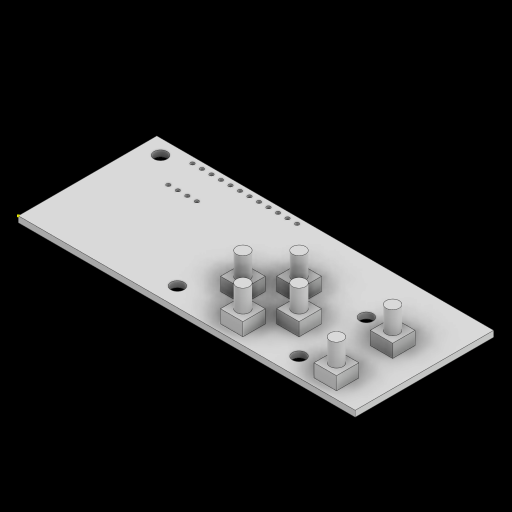
# Autodesk Inventor part: 110_PICO_Daughterboard
Saved by Autodesk Inventor 2024 (Build 280153000, 153)
## iProperties
Created: 2023-07-20
Part Number: 110_PICO_Daughterboard
Material: Generisch
Document SubType Name: Modeling
Designer: Philipp
Density: 1 g/cm^3
Appearance: Vorgabe
Author: Philipp
Autodesk Inventor part; units mm, degrees
ref_plane "YZ Plane" through (0, 0, 0) normal (1, 0, 0) x (0, 1, 0)
ref_plane "XZ Plane" through (0, 0, 0) normal (0, 1, 0) x (-1, 0, 0)
ref_plane "XY Plane" through (0, 0, 0) normal (0, 0, 1) x (1, 0, 0)
sketch "Skizze1" plane through (0, 0, 0) normal (0, 0, 1) x (1, 0, 0)
  line L0 (0, 0) -> (90, 0)
  line L1 (90, 0) -> (90, 37)
  line L2 (90, 37) -> (0, 37)
  line L3 (0, 37) -> (0, 0)
  dimension "d0" = 90
  dimension "d1" = 37
  constraints: 8 end point, 2 parallel, 1 horizontal, 1 perpendicular
  measures "d0" distance of L2.end L1.end
  measures "d1" distance of L1.end L0.end
extrude "Extrusion1" add sketch "Skizze1" against normal blind 1.6
sketch "Skizze2" plane through (0, 0, 0) normal (0, 0, 1) x (1, 0, 0)
  circle A0 centre (5, 33) radius 1.75
  circle A1 centre (37.5, 5) radius 1.75
  circle A2 centre (70, 5) radius 1.75
  circle A3 centre (70, 23) radius 1.75
  line L0 (0, 0) -> (90, 0) projected
  line L1 (0, 37) -> (0, 0) projected
  line L2 (90, 0) -> (90, 37) projected
  dimension "d4" = 3.5
  dimension "d5" = 3.5
  dimension "d6" = 3.5
  dimension "d7" = 3.5
  dimension "d8" = 33
  dimension "d9" = 5
  dimension "d10" = 37.5
  dimension "d11" = 5
  dimension "d12" = 5
  dimension "d14" = 70
  dimension "d15" = 70
  dimension "d16" = 23
  constraints: 4 centre point
  measures "d4" diameter of A0
  measures "d5" diameter of A1
  measures "d6" diameter of A2
  measures "d7" diameter of A3
  measures "d8" distance from line of L0 A0.centre
  measures "d9" distance from line of L1 A0.centre
  measures "d10" distance from line of L1 A1.centre
  measures "d11" distance from line of L0 A1.centre
  measures "d12" distance from line of L0 A2.centre
  measures "d14" distance from line of L1 A2.centre
  measures "d15" distance from line of L1 A3.centre
  measures "d16" distance from line of L0 A3.centre
extrude "Extrusion2" cut sketch "Skizze2" against normal blind 1.6
sketch "Skizze3" plane through (0, 0, 0) normal (0, 0, 1) x (1, 0, 0)
  circle A0 centre (11.152, 35.373) radius 0.5
  line L0 (0, 0) -> (90, 0) projected
  line L1 (0, 37) -> (0, 0) projected
  circle A1 centre (12.889, 27.192) radius 0.5
  dimension "d19" = 1
  dimension "d20" = 35.373
  dimension "d21" = 11.152
  dimension "d22" = 1
  dimension "d23" = 27.192
  dimension "d24" = 12.889
  constraints: 2 centre point
  measures "d19" diameter of A0
  measures "d20" distance from line of L0 A0.centre
  measures "d21" distance from line of L1 A0.centre
  measures "d22" diameter of A1
  measures "d23" distance from line of L0 A1.centre
  measures "d24" distance from line of L1 A1.centre
extrude "Extrusion3" cut sketch "Skizze3" against normal blind 1.6
pattern_linear "Rechteckige Anordnung1" count 12 spacing 2.54 along (1, 0, 0) of "Extrusion3"
sketch "Skizze4" plane through (0, 0, 0) normal (0, 0, 1) x (1, 0, 0)
  line L0 (21.549, 28.192) -> (42.329, 28.192)
  line L1 (42.329, 28.192) -> (42.329, 26.192)
  line L2 (42.329, 26.192) -> (21.549, 26.192)
  line L3 (21.549, 26.192) -> (21.549, 28.192)
  circle A0 centre (23.049, 27.192) radius 0.5 projected
  circle A1 centre (40.829, 27.192) radius 0.5 projected
  point P0 (0, 0)
  dimension "d30" = 1
  dimension "d31" = 1
  dimension "d32" = 1
  dimension "d33" = 1
  constraints: 8 end point, 2 parallel, 1 horizontal, 1 perpendicular
  measures "d30" distance edge to line of A0 L3
  measures "d31" distance edge to line of A1 L1
  measures "d32" distance from line of A0.centre L2
  measures "d33" distance from line of L0 A0.centre
extrude "Extrusion4" add sketch "Skizze4" against normal blind 1.6 contours L0 L1 L2 L3 | A0 | A1
sketch "Skizze5" plane through (0, 0, 0) normal (0, 0, 1) x (1, 0, 0)
  line L0 (0, 37) -> (0, 0) projected
  line L1 (44.5, 15.5) -> (50.5, 15.5)
  line L2 (50.5, 15.5) -> (50.5, 9.5)
  line L3 (50.5, 9.5) -> (44.5, 9.5)
  line L4 (44.5, 9.5) -> (44.5, 15.5)
  line L5 (0, 0) -> (90, 0) projected
  line L6 (52, 23) -> (58, 23)
  line L7 (58, 23) -> (58, 17)
  line L8 (58, 17) -> (52, 17)
  line L9 (52, 17) -> (52, 23)
  line L10 (52, 8) -> (58, 8)
  line L11 (58, 8) -> (58, 2)
  line L12 (58, 2) -> (52, 2)
  line L13 (52, 2) -> (52, 8)
  line L14 (59.5, 15.5) -> (65.5, 15.5)
  line L15 (65.5, 15.5) -> (65.5, 9.5)
  line L16 (65.5, 9.5) -> (59.5, 9.5)
  line L17 (59.5, 9.5) -> (59.5, 15.5)
  line L18 (77, 23) -> (83, 23)
  line L19 (83, 23) -> (83, 17)
  line L20 (83, 17) -> (77, 17)
  line L21 (77, 17) -> (77, 23)
  line L22 (77, 8) -> (83, 8)
  line L23 (83, 8) -> (83, 2)
  line L24 (83, 2) -> (77, 2)
  line L25 (77, 2) -> (77, 8)
  point P0 (44.5, 12.5)
  point P1 (47.5, 9.5)
  point P2 (55, 17)
  point P3 (52, 20)
  point P4 (52, 5)
  point P5 (55, 2)
  point P6 (62.5, 9.5)
  point P7 (59.5, 12.5)
  point P8 (83, 20)
  point P9 (80, 17)
  point P10 (83, 5)
  point P11 (80, 2)
  dimension "d34" = 1.6
  dimension "d53" = 6
  dimension "d54" = 6
  dimension "d55" = 12.5
  dimension "d56" = 47.5
  dimension "d57" = 6
  dimension "d58" = 6
  dimension "d59" = 55
  dimension "d60" = 20
  dimension "d61" = 6
  dimension "d62" = 6
  dimension "d63" = 5
  dimension "d64" = 55
  dimension "d65" = 6
  dimension "d66" = 6
  dimension "d67" = 62.5
  dimension "d68" = 12.5
  dimension "d69" = 6
  dimension "d70" = 6
  dimension "d71" = 20
  dimension "d72" = 80
  dimension "d73" = 6
  dimension "d74" = 6
  dimension "d75" = 5
  dimension "d76" = 80
  constraints: 48 end point, 12 midpoint, 12 parallel, 6 horizontal, 6 perpendicular
  measures "d53" distance of L2.end L3.end
  measures "d54" distance of L1.end L2.end
  measures "d55" distance from line of L5 point (44.5, 12.5)
  measures "d56" distance from line of point (47.5, 9.5) L0
  measures "d57" distance of L7.end L8.end
  measures "d58" distance of L6.end L7.end
  measures "d59" distance from line of L0 point (55, 17)
  measures "d60" distance from line of L5 point (52, 20)
  measures "d61" distance of L11.end L12.end
  measures "d62" distance of L10.end L11.end
  measures "d63" distance from line of L5 point (52, 5)
  measures "d64" distance from line of L0 point (55, 2)
  measures "d65" distance of L15.end L16.end
  measures "d66" distance of L14.end L15.end
  measures "d67" distance from line of L0 point (62.5, 9.5)
  measures "d68" distance from line of L5 point (59.5, 12.5)
  measures "d69" distance of L19.end L20.end
  measures "d70" distance of L18.end L19.end
  measures "d71" distance from line of L5 point (83, 20)
  measures "d72" distance from line of L0 point (80, 17)
  measures "d73" distance of L23.end L24.end
  measures "d74" distance of L22.end L23.end
  measures "d75" distance from line of L5 point (83, 5)
  measures "d76" distance from line of L0 point (80, 2)
extrude "Extrusion5" add sketch "Skizze5" along normal blind 3.5
sketch "Skizze6" plane through (0, 0, 3.5) normal (0, 0, 1) x (1, 0, 0)
  line L0 (52, 17) -> (58, 17) projected
  line L1 (58, 17) -> (58, 23) projected
  line L2 (58, 23) -> (52, 23) projected
  line L3 (52, 23) -> (52, 17) projected
  line L4 (44.5, 9.5) -> (50.5, 9.5) projected
  line L5 (50.5, 9.5) -> (50.5, 15.5) projected
  line L6 (50.5, 15.5) -> (44.5, 15.5) projected
  line L7 (44.5, 15.5) -> (44.5, 9.5) projected
  line L8 (52, 2) -> (58, 2) projected
  line L9 (58, 2) -> (58, 8) projected
  line L10 (58, 8) -> (52, 8) projected
  line L11 (52, 8) -> (52, 2) projected
  line L12 (59.5, 9.5) -> (65.5, 9.5) projected
  line L13 (65.5, 9.5) -> (65.5, 15.5) projected
  line L14 (65.5, 15.5) -> (59.5, 15.5) projected
  line L15 (59.5, 15.5) -> (59.5, 9.5) projected
  line L16 (77, 17) -> (83, 17) projected
  line L17 (83, 17) -> (83, 23) projected
  line L18 (83, 23) -> (77, 23) projected
  line L19 (77, 23) -> (77, 17) projected
  line L20 (77, 2) -> (83, 2) projected
  line L21 (83, 2) -> (83, 8) projected
  line L22 (83, 8) -> (77, 8) projected
  line L23 (77, 8) -> (77, 2) projected
  circle A0 centre (47.5, 12.5) radius 1.75
  circle A1 centre (55, 20) radius 1.75
  circle A2 centre (62.5, 12.5) radius 1.75
  circle A3 centre (55, 5) radius 1.75
  circle A4 centre (80, 5) radius 1.75
  circle A5 centre (80, 20) radius 1.75
  point P0 (0, 0)
  dimension "d79" = 3.5
  dimension "d80" = 3.5
  dimension "d81" = 3.5
  dimension "d82" = 3.5
  dimension "d83" = 3.5
  dimension "d84" = 3.5
  constraints: 6 centre point
  measures "d79" diameter of A0
  measures "d80" diameter of A1
  measures "d81" diameter of A2
  measures "d82" diameter of A3
  measures "d83" diameter of A4
  measures "d84" diameter of A5
extrude "Buttons" add sketch "Skizze6" along normal blind 6 contours A0 | A1 | A2 | A3 | A4 | A5
sketch "Skizze7" plane through (0, 0, 0) normal (0, 0, 1) x (1, 0, 0)
  point P0 (0, 0)
